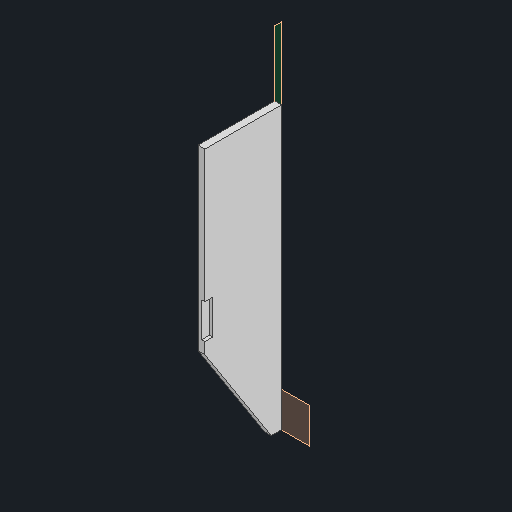
# Autodesk Inventor part: right_side
Saved by Autodesk Inventor 2023 (Build 270158000, 158)
## iProperties
Created: 2024-04-23
Part Number: right_side
Material: Generic
Document SubType Name: Modeling
Designer: szymo
Density: 1 g/cm^3
Appearance: Default
Author: szymo
Autodesk Inventor part; units mm, degrees
ref_plane "YZ Plane" through (0, 0, 0) normal (1, 0, 0) x (0, 1, 0)
ref_plane "XZ Plane" through (0, 0, 0) normal (0, 1, 0) x (-1, 0, 0)
ref_plane "XY Plane" through (0, 0, 0) normal (0, 0, 1) x (1, 0, 0)
ref_plane "Work Plane4" through (-12.2663, 62.5, -3) normal (-1, 0, 0) x (0, 0, 1)
sketch "Sketch4" plane through (-12.2663, 62.5, -3) normal (-1, 0, 0) x (0, 0, 1)
  line L0 (0, -23) -> (0, -129) projected
  line L1 (0, -129) -> (3, -129) projected
  line L2 (3, -23) -> (3, -129) projected
  line L3 (0, -23) -> (3, -23) projected
  circle A0 centre (13.5, 4.5) radius 25 projected
  line L4 (7.5, -146) -> (3, -146) projected
  line L5 (3, -146) -> (3, -150) projected
  line L6 (3, -150) -> (-0.5, -150) projected
  line L7 (-0.5, -150) -> (-0.5, -164) projected
  line L8 (-0.5, -164) -> (8.5, -150) projected
  line L9 (8.5, -150) -> (7.5, -150) projected
  line L10 (7.5, -150) -> (7.5, -146) projected
  line L11 (0, -132) -> (0, -150) projected
  line L12 (0, -150) -> (3, -150) projected
  line L13 (3, -132) -> (3, -150) projected
  line L14 (3, -107) -> (3, -129) projected
  line L15 (0, -129) -> (0, -107) projected
  line L16 (7.5, -146) -> (3, -146)
  line L17 (3, -146) -> (3, -23)
  line L18 (3, -23) -> (36.5, -23)
  line L19 (8.5, -150) -> (66.1149, -60.3768)
  line L20 (7.5, -146) -> (63.7229, -58.5421)
  line L21 (36.5, -23) -> (36.5, -100.8889)
  line L22 (36.5, -98.0889) -> (33.5, -98.0889)
  line L23 (33.5, -98.0889) -> (33.5, -82.9889)
  line L24 (33.5, -82.9889) -> (36.5, -82.9889)
  line L25 (36.5, -82.9889) -> (36.5, -98.0889)
  line L26 (0, -132) -> (3, -132) projected
  point P0 (3, -62.5)
  point P1 (38.5, 4.5)
  point P2 (3, -129)
  point P3 (3, -132)
  dimension "d4" = 25
  dimension "d5" = 2
  dimension "d9" = 2.8
  dimension "d10" = 15.1
  dimension "d11" = 3
  constraints: 20 end point, 3 horizontal, 3 parallel, 2 collinear, 2 point on line, 1 horizontal alignment, 1 perpendicular, 1 vertical, 1 other
  measures "d4" distance of point (13.5, 4.5) point (38.5, 4.5)
  measures "d5" distance from line of point (38.5, 4.5) L21
  measures "d9" distance from line of L22 L21.end
  measures "d10" distance of L22.end L23.end
  measures "d11" distance between parallel lines of L25 L23
extrude "Extrusion1" add sketch "Sketch4" against normal blind 3 contours L18 L21 L24 L23 L22 L20 L4 L13 L17 L2 | L21 L22 L23 L24
sketch "Sketch10" plane through (-9.2663, 62.5, -3) normal (1, 0, 0) x (0, 0, -1)
  line L0 (-36.5, -23) -> (-36.5, -100.8889) projected
  line L1 (-36.5, -95.8889) -> (-33, -95.8889)
  line L2 (-33, -95.8889) -> (-33, -80.7889)
  line L3 (-33, -80.7889) -> (-36.5, -80.7889)
  line L4 (-36.5, -80.7889) -> (-36.5, -95.8889)
  point P0 (-3, -62.5)
  point P1 (-36.5, -80.7889)
  dimension "d20" = 3.5
  dimension "d21" = 15.1
  dimension "d22" = 5
  constraints: 8 end point, 2 parallel, 1 horizontal, 1 perpendicular, 1 point on line
  measures "d20" distance of L3.end L2.end
  measures "d21" distance of L2.end L1.end
  measures "d22" distance of L0.end L1.start
extrude "Extrusion4" cut sketch "Sketch10" against normal blind 1.4
ref_plane "Work Plane5" through (1.7337, -83.5, -0.5885) normal (0, 0, 1) x (1, 0, 0)
body "Solid1"
